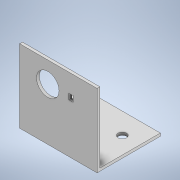
# Autodesk Inventor part: POT mount
Saved by Autodesk Inventor 2020.4 (Build 244396000, 396)
## iProperties
Created: 2022-04-16
Part Number: POT mount
Material: Generic
Document SubType Name: Modeling
Designer: Gurkin
Density: 1 g/cm^3
Appearance: Default
Author: Gurkin
Autodesk Inventor part; units mm, degrees
ref_plane "YZ Plane" through (0, 0, 0) normal (1, 0, 0) x (0, 1, 0)
ref_plane "XZ Plane" through (0, 0, 0) normal (0, 1, 0) x (-1, 0, 0)
ref_plane "XY Plane" through (0, 0, 0) normal (0, 0, 1) x (1, 0, 0)
sketch "Sketch1" plane through (0, 0, 0) normal (0, 0, 1) x (1, 0, 0)
  line L0 (0, 0) -> (55, 0)
  line L1 (55, 0) -> (55, 50)
  line L2 (55, 50) -> (0, 50)
  line L3 (0, 50) -> (0, 0)
  dimension "d3" = 55
  dimension "d4" = 50
  constraints: 8 end point, 2 parallel, 1 horizontal, 1 perpendicular
  measures "d3" distance between parallel lines of L1 L3
  measures "d4" distance between parallel lines of L0 L2
extrude "Extrusion1" add sketch "Sketch1" along normal blind 2
sketch "Sketch2" plane through (0, 0, 2) normal (0, 0, 1) x (1, 0, 0)
  circle A0 centre (20, 35) radius 8
  line L0 (0, 0) -> (55, 0) projected
  line L1 (0, 50) -> (0, 0) projected
  line L2 (35, 37) -> (38, 37)
  line L3 (38, 37) -> (38, 33)
  line L4 (38, 33) -> (35, 33)
  line L5 (35, 33) -> (35, 37)
  dimension "d2" = 16
  dimension "d5" = 35
  dimension "d6" = 20
  dimension "d7" = 15
  dimension "d8" = 4
  dimension "d9" = 3
  dimension "d10" = 2
  constraints: 8 end point, 2 parallel, 1 centre point, 1 horizontal, 1 perpendicular
  measures "d2" diameter of A0
  measures "d5" distance from line of L0 A0.centre
  measures "d6" distance from line of L1 A0.centre
  measures "d7" distance from line of L5 A0.centre
  measures "d8" distance between parallel lines of L4 L2
  measures "d9" distance between parallel lines of L5 L3
  measures "d10" distance from line of A0.centre L4
extrude "Extrusion2" cut sketch "Sketch2" against normal through all
sketch "Sketch4" plane through (0, 0, 2) normal (0, 0, 1) x (1, 0, 0)
  line L0 (0, 0) -> (55, 0)
  line L1 (55, 0) -> (55, -2)
  line L2 (55, -2) -> (0, -2)
  line L3 (0, -2) -> (0, 0)
  dimension "d13" = 2
  dimension "d14" = 55
  constraints: 8 end point, 2 parallel, 1 horizontal, 1 perpendicular
  measures "d13" distance between parallel lines of L2 L0
  measures "d14" distance between parallel lines of L3 L1
extrude "Extrusion3" add sketch "Sketch4" against normal blind 45
sketch "Sketch5" plane through (0, 0, 0) normal (0, 1, 0) x (1, 0, 0)
  circle A0 centre (12, 28) radius 3
  circle A1 centre (43, 28) radius 3
  line L0 (0, 43) -> (55, 43) projected
  line L1 (0, 0) -> (0, 43) projected
  line L2 (55, 0) -> (55, 43) projected
  dimension "d17" = 6
  dimension "d18" = 6
  dimension "d19" = 15
  dimension "d20" = 15
  dimension "d21" = 12
  dimension "d22" = 12
  constraints: 2 centre point
  measures "d17" diameter of A0
  measures "d18" diameter of A1
  measures "d19" distance from line of A0.centre L0
  measures "d20" distance from line of L0 A1.centre
  measures "d21" distance from line of L1 A0.centre
  measures "d22" distance from line of L2 A1.centre
extrude "Extrusion4" cut sketch "Sketch5" against normal through all
body "Solid1"
